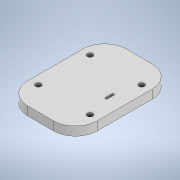
# Autodesk Inventor part: Podstawa_najwiekszy_silnik
Saved by Autodesk Inventor 2020 (Build 240168000, 168)
## iProperties
Created: 2021-03-05
Part Number: Podstawa_najwiekszy_silnik
Material: Generic
Document SubType Name: Modeling
Designer: patry
Density: 1 g/cm^3
Appearance: Default
Author: patry
Autodesk Inventor part; units mm, degrees
ref_plane "YZ Plane" through (0, 0, 0) normal (1, 0, 0) x (0, 1, 0)
ref_plane "XZ Plane" through (0, 0, 0) normal (0, 1, 0) x (-1, 0, 0)
ref_plane "XY Plane" through (0, 0, 0) normal (0, 0, 1) x (1, 0, 0)
sketch "Sketch1" plane through (0, 0, 0) normal (0, 1, 0) x (-1, 0, 0)
  line L0 (-44.8, -75) -> (-44.8, -25)
  arc A0 (-25, -5.2) -> (-44.8, -25) centre (-25, -25) ccw
  arc A1 (-44.8, -75) -> (-25, -94.8) centre (-25, -75) ccw
  circle A2 centre (10.25, -26.5) radius 2.5
  circle A3 centre (10.25, -73.5) radius 2.5
  circle A4 centre (-36.75, -73.5) radius 2.5
  circle A5 centre (-36.75, -26.5) radius 2.5
  arc A6 (18.3, -25) -> (-1.5, -5.2) centre (-1.5, -25) ccw
  arc A7 (-1.5, -94.8) -> (18.3, -75) centre (-1.5, -75) ccw
  line L1 (18.3, -25) -> (18.3, -75)
  arc A8 (-30.25, -47) -> (-32.25, -47) centre (-31.25, -47) ccw
  arc A9 (-32.25, -53) -> (-30.25, -53) centre (-31.25, -53) ccw
  line L2 (-30.25, -47) -> (-30.25, -53)
  line L3 (-32.25, -47) -> (-32.25, -53)
  line L4 (-1.5, -5.2) -> (-25, -5.2)
  line L5 (-1.5, -94.8) -> (-25, -94.8)
  point P0 (0, 0)
  point P1 (0, 0)
  point P2 (47, 5)
  point P3 (47, 93)
  point P4 (47, 95)
  point P5 (47, 25)
  point P6 (45, 25)
  point P7 (45, 75)
  point P8 (47, 75)
  point P9 (25, 5)
  point P10 (45, 25)
  point P11 (25, 95)
  point P12 (45, 75)
  dimension "d62" = 5
  dimension "d63" = 5
  dimension "d64" = 5
  dimension "d65" = 5
  dimension "d67" = 39.6
  dimension "d68" = 39.6
  constraints: 12 end point, 12 point on circle, 10 centre point, 5 tangent, 2 horizontal, 2 vertical
  measures "d62" diameter of A2
  measures "d63" diameter of A3
  measures "d64" diameter of A4
  measures "d65" diameter of A5
  measures "d67" diameter of A6
  measures "d68" diameter of A7
extrude "Extrusion6" add sketch "Sketch1" along normal blind 8
sketch "Sketch7" plane through (0, 0, 0) normal (0, -1, 0) x (1, 0, 0)
  line L0 (40.75, -28.8094) -> (36.75, -31.1188)
  line L1 (36.75, -31.1188) -> (32.75, -28.8094)
  line L2 (32.75, -28.8094) -> (32.75, -24.1906)
  line L3 (32.75, -24.1906) -> (36.75, -21.8812)
  line L4 (36.75, -21.8812) -> (40.75, -24.1906)
  line L5 (40.75, -24.1906) -> (40.75, -28.8094)
  line L6 (40.75, -75.8094) -> (36.75, -78.1188)
  line L7 (36.75, -78.1188) -> (32.75, -75.8094)
  line L8 (32.75, -75.8094) -> (32.75, -71.1906)
  line L9 (32.75, -71.1906) -> (36.75, -68.8812)
  line L10 (36.75, -68.8812) -> (40.75, -71.1906)
  line L11 (40.75, -71.1906) -> (40.75, -75.8094)
  line L12 (-6.25, -75.8094) -> (-10.25, -78.1188)
  line L13 (-10.25, -78.1188) -> (-14.25, -75.8094)
  line L14 (-14.25, -75.8094) -> (-14.25, -71.1906)
  line L15 (-14.25, -71.1906) -> (-10.25, -68.8812)
  line L16 (-10.25, -68.8812) -> (-6.25, -71.1906)
  line L17 (-6.25, -71.1906) -> (-6.25, -75.8094)
  line L18 (-6.25, -28.8094) -> (-10.25, -31.1188)
  line L19 (-10.25, -31.1188) -> (-14.25, -28.8094)
  line L20 (-14.25, -28.8094) -> (-14.25, -24.1906)
  line L21 (-14.25, -24.1906) -> (-10.25, -21.8812)
  line L22 (-10.25, -21.8812) -> (-6.25, -24.1906)
  line L23 (-6.25, -24.1906) -> (-6.25, -28.8094)
  point P0 (0, 0)
  constraints: 48 end point
extrude "Extrusion7" cut sketch "Sketch7" against normal blind 4
body "Solid4"
